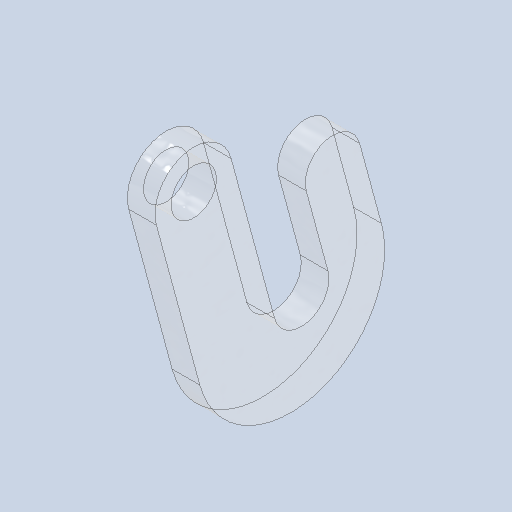
# Autodesk Inventor part: part3
Saved by Autodesk Inventor 2025.2 (Build 292293000, 293)
## iProperties
Created: 2025-02-28
Part Number: part3
Material: アクリル、クリア
Document SubType Name: Modeling
Designer: haruy
Density: 1.19 g/cm^3
Appearance: 透明 - クリア
Author: haruy
Autodesk Inventor part; units mm, degrees
ref_plane "YZ Plane" through (0, 0, 0) normal (1, 0, 0) x (0, 1, 0)
ref_plane "XZ Plane" through (0, 0, 0) normal (0, 1, 0) x (-1, 0, 0)
ref_plane "XY Plane" through (0, 0, 0) normal (0, 0, 1) x (1, 0, 0)
derived "oikon-Sketch-Base.ipt"
sketch "スケッチ1" plane through (100, 0, 0) normal (1, 0, 0) x (0, 1, 0)
  line L0 (0, 0) -> (-50, 0)
  line L1 (-50, 0) -> (-50, -5)
  line L2 (-50, -5) -> (0, -5)
  line L3 (0, -5) -> (0, 0)
  circle A0 centre (-9, -9) radius 4 construction
  circle A1 centre (-9, -9) radius 7
  line L4 (-21, 5) -> (-40, 5)
  line L5 (-40, 5) -> (-40, -5)
  line L6 (-40, -5) -> (-21, -5)
  line L7 (-21, -5) -> (-21, 5)
  line L8 (0, 8.5) -> (-50, 8.5)
  line L9 (-50, 8.5) -> (-50, 7)
  line L10 (-50, 7) -> (0, 7)
  line L11 (0, 7) -> (0, 8.5)
  line L12 (0, 18.5) -> (-50, 18.5)
  line L13 (-50, 18.5) -> (-50, 13.5)
  line L14 (-50, 13.5) -> (0, 13.5)
  line L15 (0, 13.5) -> (0, 18.5)
  line L16 (-10.8313, -2.2438) -> (-39.7865, -10.092)
  arc A2 (-29, -5) -> (-27, -5) centre (-28, -5) ccw
  line L17 (-7.1687, -15.7562) -> (-36.124, -23.6045)
  line L18 (-39.7865, -10.092) -> (-36.124, -23.6045)
  line L19 (-36.124, -23.6045) -> (-30.8918, -42.908)
  arc A3 (-36.124, -23.6045) -> (-33.5079, -33.2562) centre (-34.8159, -28.4303) ccw
  line L20 (-33.5079, -33.2562) -> (-19.0303, -29.3321)
  line L21 (-19.0303, -29.3321) -> (-16.8241, -37.4713)
  arc A4 (-16.4142, -38.9838) -> (-19.0303, -29.3321) centre (-17.7222, -34.158) ccw
  line L22 (-16.4142, -38.9838) -> (-30.8918, -42.908)
  arc A5 (-39.7865, -10.092) -> (-30.8918, -42.908) centre (-35.3391, -26.5) ccw
  line L23 (0, 0) -> (5, 0)
  line L24 (5, 0) -> (5, -5)
  line L25 (5, -5) -> (0, -5)
  line L26 (0, -5) -> (0, 0)
  line L27 (0, 18.5) -> (5, 18.5)
  line L28 (5, 18.5) -> (5, 13.5)
  line L29 (5, 13.5) -> (0, 13.5)
  line L30 (0, 13.5) -> (0, 18.5)
  line L31 (-50, 18.5) -> (-55, 18.5)
  line L32 (-55, 18.5) -> (-55, 13.5)
  line L33 (-55, 13.5) -> (-50, 13.5)
  line L34 (-50, 13.5) -> (-50, 18.5)
  line L35 (-50, 0) -> (-55, 0)
  line L36 (-55, 0) -> (-55, -5)
  line L37 (-55, -5) -> (-50, -5)
  line L38 (-50, -5) -> (-50, 0)
  circle A6 centre (-9, -9) radius 4.1
  point P0 (-14.1989, -5)
  dimension "d1" = 8.2
  measures "d1" diameter of A6
extrude "押し出し1" add sketch "スケッチ1" along normal blind 5 contours L16 A1 L2 | L2 A1 L17 L18 L16 | A1 L2 A6 | L2 A6 A1 | L18 A3 L19 A5 | L19 L20 A4 L22
